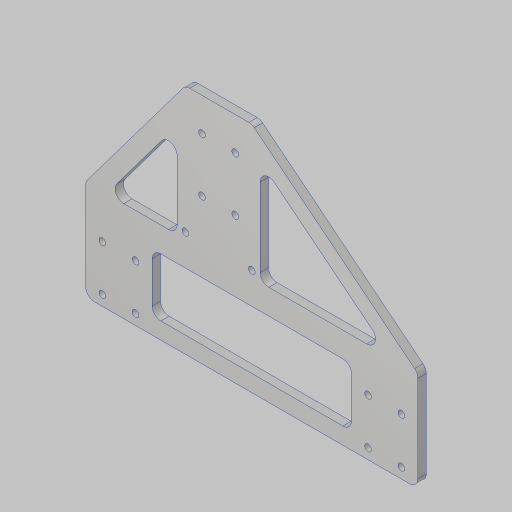
# Autodesk Inventor part: EL2-S-002
Saved by Autodesk Inventor 2023.5 (Build 275446000, 446)
## iProperties
Created: 2025-01-13
Part Number: EL2-S-002
Material: Aluminum 6061
Document SubType Name: Modeling
Designer: mavericks
Density: 2.7 g/cm^3
Appearance: Aluminum - Flat
Author: mavericks
Autodesk Inventor part; units mm, degrees
ref_plane "YZ Plane" through (0, 0, 0) normal (1, 0, 0) x (0, 1, 0)
ref_plane "XZ Plane" through (0, 0, 0) normal (0, 1, 0) x (-1, 0, 0)
ref_plane "XY Plane" through (0, 0, 0) normal (0, 0, 1) x (1, 0, 0)
sketch "Sketch1" plane through (0, 0, 0) normal (0, 0, 1) x (1, 0, 0)
  line L0 (0, 0) -> (50.8, 0) construction
  line L1 (50.8, 0) -> (50.8, 203.2) construction
  line L2 (50.8, 203.2) -> (0, 203.2) construction
  line L3 (0, 203.2) -> (0, 0) construction
  line L4 (-76.2, 0) -> (177.8, 0) construction
  line L5 (177.8, 0) -> (177.8, -76.2) construction
  line L6 (177.8, -76.2) -> (-76.2, -76.2) construction
  line L7 (-76.2, -76.2) -> (-76.2, 0) construction
  line L8 (165.1, -33.3375) -> (165.1, -68.2625) construction
  circle A0 centre (165.1, -33.3375) radius 4.7625 construction
  line L9 (174.625, -3.175) -> (-73.025, -3.175) construction
  line L10 (-73.025, -3.175) -> (-73.025, -73.025) construction
  line L11 (-73.025, -73.025) -> (174.625, -73.025) construction
  line L12 (174.625, -73.025) -> (174.625, -3.175) construction
  circle A1 centre (165.1, -68.2625) radius 4.7625 construction
  line L13 (-76.2, -76.2) -> (-76.2, 0)
  line L14 (-76.2, 0) -> (0, 101.6)
  line L15 (0, 101.6) -> (50.8, 101.6)
  line L16 (50.8, 101.6) -> (177.8, 0)
  line L17 (177.8, 0) -> (177.8, -76.2)
  line L18 (177.8, -76.2) -> (-76.2, -76.2)
  line L19 (50.8, 101.6) -> (50.8, 0) construction
  line L20 (50.8, 0) -> (177.8, 0) construction
  line L21 (0, 101.6) -> (0, 0) construction
  line L22 (0, 0) -> (-76.2, 0) construction
  line L23 (60.325, 9.525) -> (60.325, 77.7161) construction
  line L24 (50.8, 85.3361) -> (157.4701, 0)
  line L25 (145.5638, 9.525) -> (60.325, 9.525) construction
  line L26 (-60.325, 0) -> (0, 80.4333)
  line L27 (-9.525, 67.7333) -> (-9.525, 9.525) construction
  line L28 (-9.525, 9.525) -> (-53.1813, 9.525) construction
  line L29 (-60.325, 0) -> (0, 0)
  line L30 (0, 80.4333) -> (0, 0)
  line L31 (50.8, 85.3361) -> (50.8, 0)
  line L32 (50.8, 0) -> (157.4701, 0)
  line L33 (-9.525, 9.525) -> (-9.525, 0) construction
  line L34 (0, 4.7625) -> (50.8, 4.7625) construction
  line L35 (12.7, 34.925) -> (38.1, 34.925) construction
  line L36 (-6.35, 71.9667) -> (-6.35, 0)
  line L37 (57.15, 80.2561) -> (57.15, 0)
  point P0 (152.4, -50.8)
  point P1 (165.1, -50.8)
  point P2 (139.7, -68.2625)
  point P3 (139.7, -33.3375)
  point P4 (127, -50.8)
  point P5 (114.3, -68.2625)
  point P6 (114.3, -33.3375)
  point P7 (101.6, -50.8)
  point P8 (88.9, -68.2625)
  point P9 (88.9, -33.3375)
  point P10 (76.2, -50.8)
  point P11 (63.5, -68.2625)
  point P12 (63.5, -33.3375)
  point P13 (50.8, -50.8)
  point P14 (38.1, -68.2625)
  point P15 (38.1, -33.3375)
  point P16 (25.4, -50.8)
  point P17 (12.7, -68.2625)
  point P18 (12.7, -33.3375)
  point P19 (0, -50.8)
  point P20 (-12.7, -68.2625)
  point P21 (-12.7, -33.3375)
  point P22 (-25.4, -50.8)
  point P23 (-38.1, -68.2625)
  point P24 (-38.1, -33.3375)
  point P25 (-50.8, -50.8)
  point P26 (-63.5, -68.2625)
  point P27 (-63.5, -33.3375)
  point P28 (-76.2, -50.8)
  point P29 (12.7, 76.2)
  point P30 (38.1, 76.2)
  point P31 (-9.525, 4.7625)
  point P32 (25.4, 4.7625)
  point P33 (25.4, 34.925)
  dimension "d0" = 50.8
  dimension "d1" = 203.2
  dimension "d2" = 254
  dimension "d3" = 76.2
  dimension "d4" = 127
  dimension "d5" = 12.7
  dimension "d6" = 12.7
  dimension "d7" = 9.525
  dimension "d8" = 3.175
  dimension "d9" = 9.525
  dimension "d12" = 25.4
  dimension "d17" = 25.4
  dimension "d18" = 34.925
  dimension "d19" = 25.4
  dimension "d20" = 12.7
  dimension "d21" = 9.525
  dimension "d22" = 9.525
  dimension "d32" = 111.125
  dimension "d33" = 41.275
  dimension "d35" = 12.7
  dimension "d36" = 12.7
  dimension "d37" = 9.525
  dimension "d38" = 50.8
  dimension "d39" = 34.925
  dimension "d40" = 6.35
  dimension "d41" = 6.35
  constraints: 76 end point, 13 point on line, 9 collinear, 7 perpendicular, 6 horizontal alignment, 6 midpoint, 6 parallel, 5 horizontal, 4 coincident, 4 vertical alignment, 2 centre point, 1 tangent, 1 vertical, 31 other
  measures "d0" distance of L2.end L1.end
  measures "d1" distance of L1.end L0.end
  measures "d2" distance of L5.end L6.end
  measures "d3" distance of L4.end L5.end
  measures "d4" distance of L4.end L0.end
  measures "d5" horizontal distance of point (152.4, -50.8) L8.start
  measures "d6" distance from line of L5 L8.start
  measures "d7" diameter of A0
  measures "d8" distance between parallel lines of L4 L9
  measures "d9" diameter of A1
  measures "d12" distance of L8.end point (139.7, -68.262)
  measures "d17" distance from line of L15 point (12.7, 76.2)
  measures "d18" distance from line of L0 L35.start
  measures "d19" distance of point (12.7, 76.2) point (38.1, 76.2)
  measures "d20" distance from line of L3 point (12.7, 76.2)
  measures "d21" distance between parallel lines of L19 L23
  measures "d22" distance between parallel lines of L22 L28
  measures "d32" distance from line of L6 L35.start
  measures "d33" distance of L35.end point (38.1, 76.2)
  measures "d35" distance between parallel lines of L16 L24
  measures "d36" distance between parallel lines of L14 L26
  measures "d37" distance between parallel lines of L20 L25
  measures "d38" distance of L34.start L34.end
  measures "d39" distance of L8.start L8.end
  measures "d40" distance between parallel lines of L3 L36
  measures "d41" distance between parallel lines of L31 L37
extrude "Extrusion1" add sketch "Sketch1" along normal blind 6.35 contours L13 L14 L15 L16 L17 L18 | L24 L37 L32 L31 | L26 L30 L29 L36
hole "Hole1" at (165.1, -33.3375, 0) at (165.1, -68.2625, 0) at (139.7, -68.2625, 0) at (139.7, -33.3375, 0) at (-38.1, -33.3375, 0) at (-63.5, -68.2625, 0) at (-63.5, -33.3375, 0) at (12.7, 76.2, 0) at (38.1, 76.2, 0) at (38.1, 34.925, 0) at (12.7, 34.925, 0) at (0, 4.7625, 0) at (50.8, 4.7625, 0) at (-38.1, -68.2625, 0) direction (0, 0, 1) diameter 5.1054 end through all clearance for "Flat Head Machine Screw (82)" size "#10" standard "Ansi Unified Screw Threads"
fillet "Fillet1" radius 6.604 12 edges at (50.8, 101.6, 3.175) (0, 101.6, 3.175) (177.8, 0, 3.175) (-76.2, 0, 3.175) (-76.2, -76.2, 3.175) (177.8, -76.2, 3.175) (-60.325, 0, 3.175) (157.4701, 0, 3.175) (-6.35, 0, 3.175) (57.15, 0, 3.175) (57.15, 80.2561, 3.175) (-6.35, 71.9667, 3.175)
sketch "Sketch2" plane through (0, 0, 6.35) normal (0, 0, 1) x (1, 0, 0)
  line L0 (-25.4, -19.05) -> (127, -19.05)
  line L1 (127, -19.05) -> (127, -63.5)
  line L2 (127, -63.5) -> (-25.4, -63.5)
  line L3 (-25.4, -63.5) -> (-25.4, -19.05)
  arc A0 (-6.35, 52.1547) -> (-18.2372, 56.1171) centre (-12.954, 52.1547) ccw projected
  line L4 (-18.2372, 56.1171) -> (-52.4002, 10.5664) projected
  arc A1 (-52.4002, 10.5664) -> (-47.117, 0) centre (-47.117, 6.604) ccw projected
  line L5 (-47.117, 0) -> (-12.954, 0) projected
  arc A2 (-12.954, 0) -> (-6.35, 6.604) centre (-12.954, 6.604) ccw projected
  line L6 (-6.35, 6.604) -> (-6.35, 52.1547) projected
  arc A3 (57.15, 6.604) -> (63.754, 0) centre (63.754, 6.604) ccw projected
  line L7 (63.754, 0) -> (138.6435, 0) projected
  arc A4 (138.6435, 0) -> (142.769, 11.7609) centre (138.6435, 6.604) ccw projected
  line L8 (142.769, 11.7609) -> (67.8795, 71.6725) projected
  arc A5 (67.8795, 71.6725) -> (57.15, 66.5156) centre (63.754, 66.5156) ccw projected
  line L9 (57.15, 66.5156) -> (57.15, 6.604) projected
  arc A6 (3.302, 101.6) -> (-1.9812, 98.9584) centre (3.302, 94.996) ccw projected
  line L10 (3.302, 101.6) -> (48.4834, 101.6) projected
  arc A7 (52.6089, 100.1529) -> (48.4834, 101.6) centre (48.4834, 94.996) ccw projected
  line L11 (52.6089, 100.1529) -> (175.3215, 1.9828) projected
  arc A8 (177.8, -3.174) -> (175.3215, 1.9828) centre (171.196, -3.174) ccw projected
  line L12 (177.8, -3.174) -> (177.8, -69.596) projected
  arc A9 (171.196, -76.2) -> (177.8, -69.596) centre (171.196, -69.596) ccw projected
  line L13 (171.196, -76.2) -> (-69.596, -76.2) projected
  arc A10 (-76.2, -69.596) -> (-69.596, -76.2) centre (-69.596, -69.596) ccw projected
  line L14 (-76.2, -69.596) -> (-76.2, -2.2013) projected
  arc A11 (-74.8792, 1.7611) -> (-76.2, -2.2013) centre (-69.596, -2.2013) ccw projected
  line L15 (-74.8792, 1.7611) -> (-1.9812, 98.9584) projected
  circle A12 centre (50.8, 4.7625) radius 2.5527 projected
  circle A13 centre (12.7, 34.925) radius 2.5527 projected
  circle A14 centre (38.1, 76.2) radius 2.5527 projected
  circle A15 centre (-63.5, -33.3375) radius 2.5527 projected
  circle A16 centre (-38.1, -33.3375) radius 2.5527 projected
  circle A17 centre (139.7, -68.2625) radius 2.5527 projected
  circle A18 centre (165.1, -33.3375) radius 2.5527 projected
  circle A19 centre (165.1, -68.2625) radius 2.5527 projected
  circle A20 centre (139.7, -33.3375) radius 2.5527 projected
  circle A21 centre (-63.5, -68.2625) radius 2.5527 projected
  circle A22 centre (12.7, 76.2) radius 2.5527 projected
  circle A23 centre (38.1, 34.925) radius 2.5527 projected
  circle A24 centre (0, 4.7625) radius 2.5527 projected
  circle A25 centre (-38.1, -68.2625) radius 2.5527 projected
  point P0 (0, 0)
  point P1 (127, -41.275)
  dimension "d42" = 12.7
  dimension "d43" = 12.7
  dimension "d44" = 12.7
  dimension "d45" = 19.05
  constraints: 8 end point, 2 parallel, 1 horizontal, 1 midpoint, 1 perpendicular
  measures "d42" distance from line of L3 A16.centre
  measures "d43" horizontal distance of A20.centre point (127, -41.275)
  measures "d44" distance between parallel lines of L13 L2
  measures "d45" distance between parallel lines of L0 L7
extrude "Extrusion2" cut sketch "Sketch2" against normal blind 25.4 contours L0 L1 L2 L3
fillet "Fillet2" radius 6.604 4 edges at (-25.4, -63.5, 3.175) (-25.4, -19.05, 3.175) (127, -63.5, 3.175) (127, -19.05, 3.175)
equation "\"d43\" = d42"
body "Solid1"
